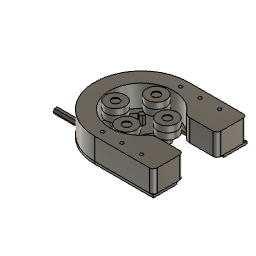
pump (Autodesk Fusion 360 design; units mm, degrees)
Autodesk Fusion 360 part; units mm, degrees
note: some values were not read from the file. Set by a fixed rule: which sketch regions a step uses.
sketch "草图1" plane through (0, 0, 0) normal (0, 0, 1) x (1, 0, 0) in component "spinner with 4 wheel v3"
  circle A0 centre (-19.1272, 19.1272) radius 4.95
  circle A1 centre (19.1272, 19.1272) radius 4.95
  circle A2 centre (19.1272, -19.1272) radius 4.95
  circle A3 centre (-19.1272, -19.1272) radius 4.95
  ellipse E0 centre (32, 0) end of major axis (47, 0) minor radius 20.5 (21.6933, 14.8943) -> (21.6933, -14.8943) ccw
  ellipse E1 centre (0, 32) end of major axis (0, 47) minor radius 20.5 (-14.8943, 21.6933) -> (14.8943, 21.6933) ccw
  line L0 (0, 41) -> (0, 70)
  line L1 (0, -47) -> (0, -70)
  ellipse E2 centre (-32, 0) end of major axis (-17, 0) minor radius 20.5 (-21.6933, -14.8943) -> (-21.6933, 14.8943) ccw
  ellipse E3 centre (0, -32) end of major axis (0, -17) minor radius 20.5 (14.8943, -21.6933) -> (-14.8943, -21.6933) ccw
  line L2 (3.25, 1.8764) -> (0, 3.7528)
  line L3 (0, 3.7528) -> (-3.25, 1.8764)
  line L4 (-3.25, 1.8764) -> (-3.25, -1.8764)
  line L5 (-3.25, -1.8764) -> (0, -3.7528)
  line L6 (0, -3.7528) -> (3.25, -1.8764)
  line L7 (3.25, -1.8764) -> (3.25, 1.8764)
  line L8 (30, -20) -> (19.1272, -19.1272)
  dimension "d5_1" = 9.9
  dimension "d6_1" = 9.9
  dimension "d7_1" = 9.9
  dimension "d8_1" = 9.9
  dimension "d9_1" = 30
  dimension "d10_1" = 41
  dimension "d15_1" = 30
  dimension "d16_1" = 41
  dimension "d17_1" = 3.25
  constraint coincident A2.centre L8.end
  measures "d5_1" diameter of A0
  measures "d6_1" diameter of A1
  measures "d7_1" diameter of A2
  measures "d8_1" diameter of A3
  measures "d9_1" distance of E0
  measures "d15_1" distance of E1
  measures "d17_1" distance of origin L7
extrude "拉伸1" add sketch "草图1" along normal blind 5 makes body 1 in component "spinner with 4 wheel v3"
sketch "草图2" plane through (0, 0, 5) normal (0, 0, 1) x (-1, 0, 0) in component "spinner with 4 wheel v3"
  line L0 (-3.25, -1.8764) -> (-3.25, 1.8764)
  line L1 (-3.25, 1.8764) -> (0, 3.7528)
  line L2 (0, 3.7528) -> (3.25, 1.8764)
  line L3 (3.25, 1.8764) -> (3.25, -1.8764)
  line L4 (3.25, -1.8764) -> (0, -3.7528)
  line L5 (0, -3.7528) -> (-3.25, -1.8764)
  ellipse E0 centre (0, 32) end of major axis (20.5, 32) minor radius 15 (-14.8943, 21.6933) -> (14.8943, 21.6933) ccw
  arc A0 (-14.8943, 21.6933) -> (-21.6933, 14.8943) centre (-19.1272, 19.1272) ccw
  ellipse E1 centre (-32, 0) end of major axis (-32, -20.5) minor radius 15 (-21.6933, -14.8943) -> (-21.6933, 14.8943) ccw
  arc A1 (-21.6933, -14.8943) -> (-14.8943, -21.6933) centre (-19.1272, -19.1272) ccw
  ellipse E2 centre (0, -32) end of major axis (20.5, -32) minor radius 15 (14.8943, -21.6933) -> (-14.8943, -21.6933) ccw
  arc A2 (14.8943, -21.6933) -> (21.6933, -14.8943) centre (19.1272, -19.1272) ccw
  ellipse E3 centre (32, 0) end of major axis (32, -20.5) minor radius 15 (21.6933, 14.8943) -> (21.6933, -14.8943) ccw
  arc A3 (21.6933, 14.8943) -> (14.8943, 21.6933) centre (19.1272, 19.1272) ccw
  circle A4 centre (-19.1272, -19.1272) radius 4.95
  circle A5 centre (19.1272, -19.1272) radius 4.95
  circle A6 centre (19.1272, 19.1272) radius 4.95
  circle A7 centre (-19.1272, 19.1272) radius 4.95
  dimension "d20_1" = 9.9
  dimension "d21_1" = 4.95
  dimension "d22_1" = 9.9
  dimension "d23_1" = 4.95
  constraint concentric A1 A4
  constraint concentric A2 A5
  constraint concentric A3 A6
  constraint concentric A0 A7
  measures "d20_1" diameter of A1
  measures "d21_1" radius of A0
  measures "d22_1" diameter of A3
  measures "d23_1" radius of A2
extrude "拉伸2" add sketch "草图2" along normal blind 7 contours A0 A7 | A3 A6 | A1 A4 | A2 A5 bodies 1 in component "spinner with 4 wheel v3"
sketch "草图3" plane through (0, 0, 5) normal (0, 0, 1) x (-1, 0, 0) in component "spinner with 4 wheel v3"
  arc A0 (-14.8943, -21.6933) -> (-21.6933, -14.8943) centre (-19.1272, -19.1272) ccw
  ellipse E0 centre (0, -32) end of major axis (20.5, -32) minor radius 15 (14.8943, -21.6933) -> (-14.8943, -21.6933) ccw
  arc A1 (21.6933, -14.8943) -> (14.8943, -21.6933) centre (19.1272, -19.1272) ccw
  ellipse E1 centre (32, 0) end of major axis (32, -20.5) minor radius 15 (21.6933, 14.8943) -> (21.6933, -14.8943) ccw
  arc A2 (14.8943, 21.6933) -> (21.6933, 14.8943) centre (19.1272, 19.1272) ccw
  ellipse E2 centre (0, 32) end of major axis (20.5, 32) minor radius 15 (-14.8943, 21.6933) -> (14.8943, 21.6933) ccw
  arc A3 (-21.6933, 14.8943) -> (-14.8943, 21.6933) centre (-19.1272, 19.1272) ccw
  ellipse E3 centre (-32, 0) end of major axis (-32, -20.5) minor radius 15 (-21.6933, -14.8943) -> (-21.6933, 14.8943) ccw
  line L0 (-3.25, -1.8764) -> (-3.25, 1.8764)
  line L1 (-3.25, 1.8764) -> (0, 3.7528)
  line L2 (0, 3.7528) -> (3.25, 1.8764)
  line L3 (3.25, 1.8764) -> (3.25, -1.8764)
  line L4 (3.25, -1.8764) -> (0, -3.7528)
  line L5 (0, -3.7528) -> (-3.25, -1.8764)
  line L6 (-3.25, -1.8764) -> (0, -3.7528)
  line L7 (0, -3.7528) -> (3.25, -1.8764)
  line L8 (3.25, -1.8764) -> (3.25, 1.8764)
  line L9 (3.25, 1.8764) -> (0, 3.7528)
  line L10 (0, 3.7528) -> (-3.25, 1.8764)
  line L11 (-3.25, 1.8764) -> (-3.25, -1.8764)
extrude "拉伸3" add sketch "草图3" against normal blind 2 contours L0 L1 L2 L3 L4 L5 L6 L7 L8 L9 L10 L11 bodies 1 in component "spinner with 4 wheel v3"
sketch "草图4" plane through (0, 0, 5) normal (0, 0, 1) x (-1, 0, 0) in component "spinner with 4 wheel v3"
  arc A0 (-14.8943, -21.6933) -> (-21.6933, -14.8943) centre (-19.1272, -19.1272) ccw
  ellipse E0 centre (0, -32) end of major axis (20.5, -32) minor radius 15 (14.8943, -21.6933) -> (-14.8943, -21.6933) ccw
  arc A1 (21.6933, -14.8943) -> (14.8943, -21.6933) centre (19.1272, -19.1272) ccw
  ellipse E1 centre (32, 0) end of major axis (32, -20.5) minor radius 15 (21.6933, 14.8943) -> (21.6933, -14.8943) ccw
  arc A2 (14.8943, 21.6933) -> (21.6933, 14.8943) centre (19.1272, 19.1272) ccw
  ellipse E2 centre (0, 32) end of major axis (20.5, 32) minor radius 15 (-14.8943, 21.6933) -> (14.8943, 21.6933) ccw
  arc A3 (-21.6933, 14.8943) -> (-14.8943, 21.6933) centre (-19.1272, 19.1272) ccw
  ellipse E3 centre (-32, 0) end of major axis (-32, -20.5) minor radius 15 (-21.6933, -14.8943) -> (-21.6933, 14.8943) ccw
  circle A4 centre (0, 0) radius 2
  constraint coincident A4.centre origin
extrude "拉伸4" add sketch "草图4" along normal blind 15 contours A4 bodies 1 in component "spinner with 4 wheel v3"
sketch "草图5" plane through (0, 0, 0) normal (0, 0, 1) x (1, 0, 0) in component "spinner with 4 wheel v3"
extrude "拉伸5" add 1 faces at (1.0833, -0.6255, 3) along direction (0, 0, -1) blind 3 on bodies 1 bodies 1 in component "spinner with 4 wheel v3"
sketch "草图6" plane through (0, 0, 0) normal (0, 0, 1) x (1, 0, 0) in component "spinner with 4 wheel v3"
  line L0 (-3.2, -1.8475) -> (0, -3.695)
  line L1 (0, -3.695) -> (3.2, -1.8475)
  line L2 (3.2, -1.8475) -> (3.2, 1.8475)
  line L3 (3.2, 1.8475) -> (0, 3.695)
  line L4 (0, 3.695) -> (-3.2, 1.8475)
  line L5 (-3.2, 1.8475) -> (-3.2, -1.8475)
  dimension "d32_1" = 3.2
  measures "d32_1" distance of origin L5
extrude "拉伸6" cut sketch "草图6" along normal blind 22 bodies 1 in component "spinner with 4 wheel v3"
sketch "草图7" plane through (0, 0, 0) normal (1, 0, 0) x (0, 1, 0) in component "spinner with 4 wheel v3"
extrude "拉伸7" cut 4 faces at (18.1573, 20.0862, 12) (16.979, -18.0927, 12) (-17.5166, -19.4446, 12) (-20.5586, 20.6052, 12) along direction (0, 0, -1) blind 12 on bodies 1 bodies 1 in component "spinner with 4 wheel v3"
sketch "草图8" plane through (0, 0, 5) normal (0, 0, 1) x (-1, 0, 0) in component "spinner with 4 wheel v3"
  arc A0 (-14.8943, -21.6933) -> (-21.6933, -14.8943) centre (-19.1272, -19.1272) ccw
  ellipse E0 centre (0, -32) end of major axis (20.5, -32) minor radius 15 (14.8943, -21.6933) -> (-14.8943, -21.6933) ccw
  arc A1 (21.6933, -14.8943) -> (14.8943, -21.6933) centre (19.1272, -19.1272) ccw
  ellipse E1 centre (32, 0) end of major axis (32, -20.5) minor radius 15 (21.6933, 14.8943) -> (21.6933, -14.8943) ccw
  arc A2 (14.8943, 21.6933) -> (21.6933, 14.8943) centre (19.1272, 19.1272) ccw
  ellipse E2 centre (0, 32) end of major axis (20.5, 32) minor radius 15 (-14.8943, 21.6933) -> (14.8943, 21.6933) ccw
  arc A3 (-21.6933, 14.8943) -> (-14.8943, 21.6933) centre (-19.1272, 19.1272) ccw
  ellipse E3 centre (-32, 0) end of major axis (-32, -20.5) minor radius 15 (-21.6933, -14.8943) -> (-21.6933, 14.8943) ccw
  circle A4 centre (-19.1272, 19.1272) radius 5
  circle A5 centre (-19.1272, -19.1272) radius 5
  circle A6 centre (19.1272, 19.1272) radius 5
  circle A7 centre (19.1272, -19.1272) radius 5
  line L0 (3.2, -1.8475) -> (0, -3.695)
  line L1 (0, -3.695) -> (-3.2, -1.8475)
  line L2 (-3.2, -1.8475) -> (-3.2, 1.8475)
  line L3 (-3.2, 1.8475) -> (0, 3.695)
  line L4 (0, 3.695) -> (3.2, 1.8475)
  line L5 (3.2, 1.8475) -> (3.2, -1.8475)
  dimension "d37" = 4.95
  dimension "d38" = 4.95
  dimension "d39" = 4.95
  dimension "d40" = 4.95
  dimension "d41" = 10
  dimension "d42" = 10
  dimension "d43" = 10
  dimension "d44" = 10
  constraint concentric A3 A4
  constraint concentric A0 A5
  constraint concentric A2 A6
  constraint concentric A1 A7
  measures "d37" radius of A3
  measures "d38" radius of A0
  measures "d39" radius of A1
  measures "d40" radius of A2
  measures "d41" diameter of A4
  measures "d42" diameter of A5
  measures "d43" diameter of A6
  measures "d44" diameter of A7
extrude "拉伸8" add sketch "草图8" along normal blind -5 and the other way blind -7 contours A0 E0 E3 A5 | A0 E0 E3 A5 | E0 A1 E1 A7 | E0 A1 E1 A7 | E2 A3 E3 A4 | E2 A3 E3 A4 | E1 A2 E2 A6 | E1 A2 E2 A6 bodies 1 in component "spinner with 4 wheel v3"
extrude "拉伸9" add 4 faces at (20.5783, 17.6971, 12) (-17.6037, 17.7136, 12) (-20.6618, -20.4674, 12) (18.5183, -20.4625, 12) along direction (0, 0, 1) blind 8 on bodies 1 bodies 1 in component "spinner with 4 wheel v3"
extrude "拉伸10" add 1 faces at (9.8129, -9.3621, 0) along direction (0, 0, -1) blind 5 on bodies 1 bodies 1 in component "spinner with 4 wheel v3"
sketch "草图1 (2)" plane through (0, 0, 0) normal (1, 0, 0) x (0, 1, 0) in component "thicker and extrusion spinner v2"
sketch "草图1 (3)" plane through (0, 0, 0) normal (0, 0, 1) x (1, 0, 0) in component "wheel v2"
  circle A0 centre (0, 0) radius 4.95
  circle A1 centre (0, 0) radius 12.5
  dimension "d3_2" = 9.9
  dimension "d4_2" = 25
  constraint concentric A0 A1
  measures "d3_2" diameter of A0
  measures "d4_2" diameter of A1
extrude "拉伸1'" add sketch "草图1 (3)" along normal blind 8 separate body makes body 2 in component "wheel v2"
sketch "草图1 (4)" plane through (0, 0, 0) normal (0, 0, 1) x (1, 0, 0) in component "wheel v2 (1)"
  circle A0 centre (0, 0) radius 4.95
  circle A1 centre (0, 0) radius 12.5
  dimension "d3_3" = 9.9
  dimension "d4_3" = 25
  constraint concentric A0 A1
  measures "d3_3" diameter of A0
  measures "d4_3" diameter of A1
extrude "拉伸1''" add sketch "草图1 (4)" along normal blind 8 separate body makes body 3 in component "wheel v2 (1)"
sketch "草图1 (5)" plane through (0, 0, 0) normal (0, 0, 1) x (1, 0, 0) in component "wheel v2 (2)"
  circle A0 centre (0, 0) radius 4.95
  circle A1 centre (0, 0) radius 12.5
  dimension "d3_4" = 9.9
  dimension "d4_4" = 25
  constraint concentric A0 A1
  measures "d3_4" diameter of A0
  measures "d4_4" diameter of A1
extrude "拉伸1'''" add sketch "草图1 (5)" along normal blind 8 separate body makes body 4 in component "wheel v2 (2)"
sketch "草图1 (6)" plane through (0, 0, 0) normal (0, 0, 1) x (1, 0, 0) in component "wheel v2 (3)"
  circle A0 centre (0, 0) radius 4.95
  circle A1 centre (0, 0) radius 12.5
  dimension "d3" = 9.9
  dimension "d4" = 25
  constraint concentric A0 A1
  measures "d3" diameter of A0
  measures "d4" diameter of A1
extrude "拉伸1''''" add sketch "草图1 (6)" along normal blind 8 separate body makes body 5 in component "wheel v2 (3)"
sketch "草图1 (7)" plane through (0, 0, 0) normal (0, 0, 1) x (1, 0, 0) in component "wheel v2 (4)"
  circle A0 centre (0, 0) radius 4.95
  circle A1 centre (0, 0) radius 12.5
  dimension "d3_5" = 9.9
  dimension "d4_5" = 25
  constraint concentric A0 A1
  measures "d3_5" diameter of A0
  measures "d4_5" diameter of A1
extrude "拉伸1'''''" add sketch "草图1 (7)" along normal blind 8 separate body makes body 6 in component "wheel v2 (4)"
sketch "草图1 (8)" plane through (0, 0, 0) normal (0, 0, 1) x (1, 0, 0) in component "wheel v2 (5)"
  circle A0 centre (0, 0) radius 4.95
  circle A1 centre (0, 0) radius 12.5
  dimension "d3_6" = 9.9
  dimension "d4_6" = 25
  constraint concentric A0 A1
  measures "d3_6" diameter of A0
  measures "d4_6" diameter of A1
extrude "拉伸1''''''" add sketch "草图1 (8)" along normal blind 8 separate body makes body 7 in component "wheel v2 (5)"
sketch "草图1 (9)" plane through (0, 0, 0) normal (0, 0, 1) x (1, 0, 0) in component "wheel v2 (6)"
  circle A0 centre (0, 0) radius 4.95
  circle A1 centre (0, 0) radius 12.5
  dimension "d3_7" = 9.9
  dimension "d4_7" = 25
  constraint concentric A0 A1
  measures "d3_7" diameter of A0
  measures "d4_7" diameter of A1
extrude "拉伸1'''''''" add sketch "草图1 (9)" along normal blind 8 separate body makes body 8 in component "wheel v2 (6)"
sketch "草图1 (10)" plane through (0, 0, 0) normal (0, 0, 1) x (1, 0, 0) in component "wheel v2 (7)"
  circle A0 centre (0, 0) radius 4.95
  circle A1 centre (0, 0) radius 12.5
  dimension "d3_8" = 9.9
  dimension "d4_8" = 25
  constraint concentric A0 A1
  measures "d3_8" diameter of A0
  measures "d4_8" diameter of A1
extrude "拉伸1''''''''" add sketch "草图1 (10)" along normal blind 8 separate body makes body 9 in component "wheel v2 (7)"
sketch "草图1 (11)" plane through (0, 0, 0) normal (0, 0, 1) x (1, 0, 0) in component "key v1"
  line L0 (-100, 50) -> (0, 50)
  arc A0 (10, 40) -> (0, 50) centre (0, 40) ccw
  line L1 (10, 40) -> (10, 0)
  line L2 (10, 0) -> (10, -1.2961)
  dimension "d1" = 100
  constraint horizontal L0
  constraint tangent L0 A0
  constraint tangent A0 L1
  constraint vertical L1
  constraint parallel L1 L2
  measures "d1" distance of L0.start L0.end
ref_plane "工作平面1" through (-100, 50, 0) normal (1, 0, 0) x (0, 1, 0) in component "key v1"
sketch "草图2 (2)" plane through (-100, 0, 0) normal (1, 0, 0) x (0, 1, 0) in component "key v1"
  line L0 (47.0037, -1.7384) -> (50.0073, -3.4641)
  line L1 (50.0073, -3.4641) -> (53.0036, -1.7257)
  line L2 (53.0036, -1.7257) -> (52.9963, 1.7384)
  line L3 (52.9963, 1.7384) -> (49.9927, 3.4641)
  line L4 (49.9927, 3.4641) -> (46.9964, 1.7257)
  line L5 (46.9964, 1.7257) -> (47.0037, -1.7384)
  point P0 (50, 0)
  dimension "d3_9" = 3
  measures "d3_9" distance of P0 L5
sweep "扫掠1" add profiles "草图2 (2)" path "草图1 (11)" along L0 A0 L1 L2 section 1 separate body makes body 10 in component "key v1"
sketch "草图1 (12)" plane through (0, 0, 0) normal (0, 0, 1) x (1, 0, 0) in component "case1 v8"
  line L0 (0, 60) -> (70, 60)
  line L1 (75, 55) -> (75, 40)
  line L2 (75, -40) -> (75, -55)
  line L3 (70, -60) -> (0, -60)
  arc A0 (0, 60) -> (0, -60) centre (0, 0) ccw
  circle A1 centre (0, -50) radius 2.1 construction
  circle A2 centre (25, -50) radius 2.1 construction
  circle A3 centre (50, -50) radius 2.1 construction
  circle A4 centre (0, 50) radius 2.1 construction
  circle A5 centre (25, 50) radius 2.1 construction
  circle A6 centre (50, 50) radius 2.1 construction
  circle A7 centre (50, 50) radius 2.1
  circle A8 centre (25, 50) radius 2.1
  circle A9 centre (0, 50) radius 2.1
  circle A10 centre (50, -50) radius 2.1
  circle A11 centre (25, -50) radius 2.1
  circle A12 centre (0, -50) radius 2.1
  arc A13 (32.3364, 25.2063) -> (32.3364, -25.2063) centre (0, 0) ccw
  line L4 (40.2233, 21.3542) -> (70, 21.3542)
  line L5 (75, 26.3542) -> (75, 40)
  line L6 (40.2233, -21.3542) -> (70, -21.3542)
  line L7 (75, -26.3542) -> (75, -40)
  arc A14 (40.2233, -21.3542) -> (32.3364, -25.2063) centre (40.2233, -31.3542) ccw
  arc A15 (32.3364, 25.2063) -> (40.2233, 21.3542) centre (40.2233, 31.3542) ccw
  arc A16 (75, 55) -> (70, 60) centre (70, 55) ccw
  arc A17 (70, 21.3542) -> (75, 26.3542) centre (70, 26.3542) ccw
  arc A18 (75, -26.3542) -> (70, -21.3542) centre (70, -26.3542) ccw
  arc A19 (70, -60) -> (75, -55) centre (70, -55) ccw
  point P0 (75, 60)
  dimension "d2" = 75
  dimension "d41_1" = 4.2
  dimension "d42_1" = 4.2
  dimension "d43_1" = 4.2
  dimension "d44_1" = 4.2
  dimension "d45_1" = 4.2
  dimension "d46_1" = 4.2
  dimension "d55_1" = 82
  dimension "d56_1" = 10
  dimension "d57_1" = 10
  dimension "d58_1" = 5
  constraint coincident A0.centre A13.centre
  constraint horizontal L0
  constraint vertical L1
  constraint vertical L2
  constraint horizontal L3
  constraint concentric A6 A7
  constraint concentric A5 A8
  constraint concentric A4 A9
  constraint concentric A3 A10
  constraint concentric A2 A11
  constraint concentric A1 A12
  constraint horizontal L4
  constraint vertical L5
  constraint horizontal L6
  constraint vertical L7
  constraint tangent A13 A14
  constraint tangent L6 A14
  constraint tangent A13 A15
  constraint tangent L4 A15
  constraint coincident P0 L0
  constraint coincident P0 L1
  constraint tangent L0 A16
  constraint tangent L1 A16
  constraint tangent L4 A17
  constraint tangent L5 A17
  constraint equal A16 A17
  constraint tangent L6 A18
  constraint tangent L7 A18
  constraint equal A16 A18
  constraint tangent L2 A19
  constraint tangent L3 A19
  constraint equal A16 A19
  measures "d2" distance of L0.start P0
  measures "d41_1" diameter of A1
  measures "d42_1" diameter of A2
  measures "d43_1" diameter of A3
  measures "d44_1" diameter of A4
  measures "d45_1" diameter of A5
  measures "d46_1" diameter of A6
  measures "d55_1" diameter of A13
  measures "d56_1" radius of A14
  measures "d57_1" radius of A15
  measures "d58_1" radius of A16
extrude "拉伸5'" add sketch "草图1 (12)" along normal blind 4 separate body makes body 11 in component "case1 v8"
extrude "Extrude4" [suppressed] in component "case1 v8"
extrude "Extrude3" [suppressed] in component "case1 v8"
extrude "拉伸6'" add sketch "草图1 (12)" along normal blind 16 and the other way blind 8 bodies 11 in component "case1 v8"
extrude "拉伸7'" add 1 faces at (53.5553, 30.2185, 16) along direction (0, 0, 1) blind 4 on bodies 11 bodies 11 in component "case1 v8"
sketch "草图1 (13)" plane through (0, 0, 0) normal (0, 0, 1) x (1, 0, 0) in component "case2 v7"
  line L0 (0, 60) -> (75, 60)
  line L1 (75, 60) -> (75, 30)
  line L2 (75, 30) -> (0, 30)
  line L3 (0, -60) -> (75, -60)
  line L4 (75, -60) -> (75, -30)
  line L5 (75, -30) -> (0, -30)
  arc A0 (0, 60) -> (0, -60) centre (0, 0) ccw
  arc A1 (0, 30) -> (0, -30) centre (0, 0) ccw
  circle A2 centre (0, 50) radius 2.1
  circle A3 centre (25, 50) radius 2.1
  circle A4 centre (50, 50) radius 2.1
  circle A5 centre (0, -50) radius 2.1
  circle A6 centre (25, -50) radius 2.1
  circle A7 centre (50, -50) radius 2.1
  dimension "d1_2" = 4.2
  dimension "d2_3" = 4.2
  dimension "d3_10" = 4.2
  dimension "d4_10" = 4.2
  dimension "d5_10" = 4.2
  dimension "d6_10" = 4.2
  constraint coincident A0.centre A1.centre
  constraint concentric A0 A1
  constraint horizontal L0
  constraint vertical L1
  constraint horizontal L2
  constraint horizontal L3
  constraint vertical L4
  constraint horizontal L5
  measures "d1_2" diameter of A2
  measures "d2_3" diameter of A3
  measures "d3_10" diameter of A4
  measures "d4_10" diameter of A5
  measures "d5_10" diameter of A6
  measures "d6_10" diameter of A7
extrude "拉伸1'''''''''" add sketch "草图1 (13)" along normal blind 3 separate body makes body 12 in component "case2 v7"
sketch "草图2 (3)" plane through (0, 0, 0) normal (0, 1, 0) x (1, 0, 0) in component "case2 v7"
sketch "草图3 (2)" plane through (0, 0, 0) normal (0, 0, 1) x (1, 0, 0) in component "case2 v7"
component "thicker and extrusion spinner v2" placed x (1, 0, 0) y (0, 1, 0) z (0, 0, 1) at (0, 0, 0)
component "wheel v2" placed x (0.867078, -0.498173, 0) y (0.498173, 0.867078, 0) z (0, 0, 1) at (7.0566, -26.3444, 4.0688)
component "wheel v2 (1)" placed x (-0.498173, -0.867078, 0) y (0.867078, -0.498173, 0) z (0, 0, 1) at (7.0566, -26.3444, 12.0688)
component "wheel v2 (2)" placed x (0.867078, -0.498173, 0) y (0.498173, 0.867078, 0) z (0, 0, 1) at (26.114, 6.8252, 4.0688)
component "wheel v2 (3)" placed x (-0.498173, -0.867078, 0) y (0.867078, -0.498173, 0) z (0, 0, 1) at (26.114, 6.8252, 12.0688)
component "wheel v2 (4)" placed x (0.867078, -0.498173, 0) y (0.498173, 0.867078, 0) z (0, 0, 1) at (-26.113, -7.2871, 4.0688)
component "wheel v2 (5)" placed x (0.867078, -0.498173, 0) y (0.498173, 0.867078, 0) z (0, 0, 1) at (-26.113, -7.2871, 12.0688)
component "wheel v2 (6)" placed x (0.867078, -0.498173, 0) y (0.498173, 0.867078, 0) z (0, 0, 1) at (-7.0556, 25.8825, 4.0688)
component "wheel v2 (7)" placed x (0.867078, -0.498173, 0) y (0.498173, 0.867078, 0) z (0, 0, 1) at (-7.0556, 25.8825, 12.0688)
component "key v1" placed x (1, 0, 0) y (0, 0, -1) z (0, 1, 0) at (-10, 0, 13.7039)
component "case1 v8" placed x (1, 0, 0) y (0, 1, 0) z (0, 0, 1) at (0, 0, 0)
component "case2 v7" placed x (1, 0, 0) y (0, 1, 0) z (0, 0, 1) at (0, 0, -11)
component "spinner with 4 wheel v3" placed x (0.498173, 0.867078, 0) y (-0.867078, 0.498173, 0) z (0, 0, 1) at (0.0005, -0.2309, -0.9312) in component "thicker and extrusion spinner v2"
